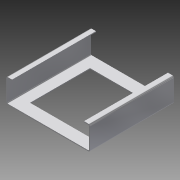
# Autodesk Inventor part: DishFanMetal
Saved by Autodesk Inventor 2014 (Build 180170000, 170)
## iProperties
Created: 2015-05-01
Part Number: DishFanMetal
Material: Generic
Document SubType Name: Sheet Metal
Designer: Owner
Density: 1 g/cm^3
Sheet Metal Rule: Default
Appearance: Aluminum - Polished
Author: Owner
Autodesk Inventor part; units mm, degrees
ref_plane "YZ Plane" through (0, 0, 0) normal (1, 0, 0) x (0, 1, 0)
ref_plane "XZ Plane" through (0, 0, 0) normal (0, 1, 0) x (-1, 0, 0)
ref_plane "XY Plane" through (0, 0, 0) normal (0, 0, 1) x (1, 0, 0)
sketch "Sketch1" plane through (0, 0, 0) normal (0, 1, 0) x (-1, 0, 0)
  line L0 (-46.7054, 45.2992) -> (53.2946, 45.2992)
  line L1 (53.2946, 45.2992) -> (53.2946, -54.7008)
  line L2 (53.2946, -54.7008) -> (-46.7054, -54.7008)
  line L3 (-46.7054, -54.7008) -> (-46.7054, 45.2992)
  line L4 (73.2946, -74.7008) -> (-66.7054, -74.7008)
  line L5 (-66.7054, -74.7008) -> (-66.7054, 65.2992)
  line L6 (-66.7054, 65.2992) -> (73.2946, 65.2992)
  line L7 (73.2946, 65.2992) -> (73.2946, -74.7008)
  point P0 (0, 0)
  dimension "d0" = 100
  dimension "d1" = 100
  dimension "d2" = 140
  dimension "d3" = 140
  dimension "d4" = 20
  dimension "d5" = 20
  measures "d0" distance of L0.start L0.end
  measures "d1" distance of L0.end L1.end
  measures "d2" distance of L5.end L6.end
  measures "d3" distance of L6.end L4.start
  measures "d4" distance between parallel lines of L6 L0
  measures "d5" distance between parallel lines of L7 L1
extrude "Plate1" add sketch "Sketch1" along normal blind 1.5875
sketch "Sketch2" plane through (65.1179, 0, -74.7008) normal (1, 0, 0) x (0, 1, 0)
  line L0 (0, 140) -> (0, 0)
  line L1 (0, 0) -> (40, 0)
  line L2 (40, 0) -> (40, 140)
  line L3 (40, 140) -> (0, 140)
  constraints: 6 end point, 1 horizontal, 1 perpendicular, 1 vertical
edge flange "Flange1" height 40 angle 90 thickness 1.5875 bend radius 1.5875 thickness toward (1, 0, 0) relief straight relief width 1.5875 relief depth 0.7937 edges at (66.7054, 1.5875, -4.7008) wall of the first edge with corners at (65.1179, 0, 65.2992) (65.1179, 0, -74.7008) (65.1179, 40, -74.7008) (65.1179, 40, 65.2992)
bend "Bend1"
corner "Corner1"
sketch "Sketch3" plane through (-71.7071, 0, 65.2992) normal (-1, 0, 0) x (0, -1, 0)
  line L0 (0, -140) -> (0, 0)
  line L1 (0, 0) -> (-40, 0)
  line L2 (-40, 0) -> (-40, -140)
  line L3 (-40, -140) -> (0, -140)
  constraints: 6 end point, 1 horizontal, 1 perpendicular, 1 vertical
edge flange "Flange2" height 40 angle 90 thickness 1.5875 bend radius 1.5875 thickness toward (-1, 0, 0) relief straight relief width 1.5875 relief depth 0.7937 edges at (-73.2946, 1.5875, -4.7008) wall of the first edge with corners at (-71.7071, 0, -74.7008) (-71.7071, 0, 65.2992) (-71.7071, 40, 65.2992) (-71.7071, 40, -74.7008)
bend "Bend2"
corner "Corner2"
sketch "Sketch4" plane through (-73.2946, 38.4125, 65.2992) normal (0, 1, 0) x (-1, 0, 0)
  line L0 (0, -140) -> (0, 0)
  line L1 (0, 0) -> (-10, 0)
  line L2 (-10, 0) -> (-10, -140)
  line L3 (-10, -140) -> (0, -140)
  constraints: 6 end point, 1 horizontal, 1 perpendicular, 1 vertical
edge flange "Flange3" height 10 angle 90 thickness 1.5875 bend radius 1.5875 thickness toward (0, 1, 0) relief straight relief width 1.5875 relief depth 0.7937 edges at (-71.7071, 40, -4.7008) wall of the first edge with corners at (-73.2946, 38.4125, -74.7008) (-73.2946, 38.4125, 65.2992) (-63.2946, 38.4125, 65.2992) (-63.2946, 38.4125, -74.7008)
bend "Bend3"
corner "Corner3"
sketch "Sketch5" plane through (66.7054, 38.4125, -74.7008) normal (0, 1, 0) x (-1, 0, 0)
  line L0 (0, 140) -> (0, 0)
  line L1 (0, 0) -> (10, 0)
  line L2 (10, 0) -> (10, 140)
  line L3 (10, 140) -> (0, 140)
  constraints: 6 end point, 1 horizontal, 1 perpendicular, 1 vertical
edge flange "Flange4" height 10 angle 90 thickness 1.5875 bend radius 1.5875 thickness toward (0, 1, 0) relief straight relief width 1.5875 relief depth 0.7937 edges at (65.1179, 40, -4.7008) wall of the first edge with corners at (66.7054, 38.4125, 65.2992) (66.7054, 38.4125, -74.7008) (56.7054, 38.4125, -74.7008) (56.7054, 38.4125, 65.2992)
bend "Bend4"
corner "Corner4"
equation "\"d7\" = BendReliefWidth"
equation "\"d8\" = BendReliefDepth"
equation "\"d9\" = MinimumRemnant"
equation "\"d10\" = BendRadius"
equation "\"d13\" = BendRadius"
equation "\"d14\" = CornerReliefSize"
equation "\"d15\" = GapSize"
equation "\"d16\" = JacobiRadiusSize"
equation "\"d17\" = BendReliefWidth"
equation "\"d18\" = BendReliefDepth"
equation "\"d19\" = MinimumRemnant"
equation "\"d20\" = BendRadius"
equation "\"d23\" = BendRadius"
equation "\"d24\" = CornerReliefSize"
equation "\"d25\" = GapSize"
equation "\"d26\" = JacobiRadiusSize"
equation "\"d27\" = BendReliefWidth"
equation "\"d28\" = BendReliefDepth"
equation "\"d29\" = MinimumRemnant"
equation "\"d30\" = BendRadius"
equation "\"d33\" = BendRadius"
equation "\"d34\" = CornerReliefSize"
equation "\"d35\" = GapSize"
equation "\"d36\" = JacobiRadiusSize"
equation "\"d37\" = BendReliefWidth"
equation "\"d38\" = BendReliefDepth"
equation "\"d39\" = MinimumRemnant"
equation "\"d40\" = BendRadius"
equation "\"d43\" = BendRadius"
equation "\"d44\" = CornerReliefSize"
equation "\"d45\" = GapSize"
equation "\"d46\" = JacobiRadiusSize"
equation "\"BendRadius\" = Thickness"
equation "\"BendReliefWidth\" = Thickness"
equation "\"BendReliefDepth\" = 0.5 * Thickness"
equation "\"CornerReliefSize\" = 4 * Thickness"
equation "\"MinimumRemnant\" = 2 * Thickness"
equation "\"TransitionRadius\" = BendRadius"
equation "\"JacobiRadiusSize\" = BendRadius"
equation "\"GapSize\" = Thickness"
equation "\"d6\" = BendRadius"
equation "\"Thickness\" = 1.5875"
body "Solid1"
